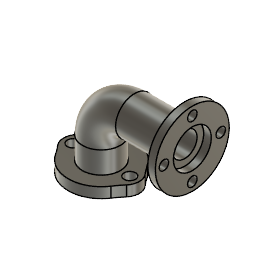
MaRS_Q5_c (Autodesk Fusion 360 design; units mm, degrees)
part number: 2026-05-28-18-50-45-195
Autodesk Fusion 360 part; units mm, degrees
sketch "Sketch1" plane through (0, 0, 0) normal (1, 0, 0) x (0, 1, 0)
sketch "Sketch2" plane through (0, 0, 0) normal (0, 0, 1) x (1, 0, 0)
  circle A0 through (-62, 0, -40) (-81.5, 11.2583, -40) (-81.5, -11.2583, -40)
  arc A1 through (-104.26, -19.2055, -40) (-75, -35, -40) (-45.74, -19.2055, -40)
  arc A2 through (-45.74, 19.2055, -40) (-75, 35, -40) (-104.26, 19.2055, -40)
  arc A3 through (-38.6429, -9.7987, -40) (-35, 0, -40) (-38.6429, 9.7987, -40)
  arc A4 through (-111.0884, 10.1122, -40) (-114.8217, 0, -40) (-111.0884, -10.1122, -40)
  circle A5 through (-55, 0, -40) (-85, 17.3205, -40) (-85, -17.3205, -40)
  arc A6 through (-111.0884, 10.1122, -40) (-107.5304, 14.5508, -40) (-104.26, 19.2055, -40)
  arc A7 through (-104.26, -19.2055, -40) (-107.5304, -14.5508, -40) (-111.0884, -10.1122, -40)
  arc A8 through (-38.6429, -9.7987, -40) (-42.3455, -14.3859, -40) (-45.74, -19.2055, -40)
  arc A9 through (-45.74, 19.2055, -40) (-42.3455, 14.3859, -40) (-38.6429, 9.7987, -40)
  circle A10 through (-39, 0, -40) (-48, 5.1962, -40) (-48, -5.1962, -40)
  circle A11 through (-99, 0, -40) (-108, 5.1962, -40) (-108, -5.1962, -40)
  dimension "d59" = 12
  dimension "d60" = 12
sketch "Sketch3" plane through (0, 0, 0) normal (0, 1, 0) x (1, 0, 0)
sketch "Sketch4" plane through (0, 0, 0) normal (0, 0, 1) x (1, 0, 0)
sketch "Sketch5" plane through (0, 0, 0) normal (0, 1, 0) x (1, 0, 0)
  line L0 (-75, 40) -> (-75, 17)
  line L1 (-40, -18) -> (13, -18)
  arc A0 (-75, 17) -> (-40, -18) centre (-40, 17) ccw
  line L2 (-95, 37.5) -> (-95, 17)
  arc A1 (-95, 17) -> (-40, -38) centre (-40, 17) ccw
  line L3 (-40, -38) -> (10.5, -38)
  line L4 (-75, 40) -> (-75, 17)
  arc A2 (-75, 17) -> (-40, -18) centre (-40, 17) ccw
  line L5 (-40, -18) -> (13, -18)
  line L6 (-55, 37.5) -> (-55, 17)
  arc A3 (-55, 17) -> (-40, 2) centre (-40, 17) ccw
  line L7 (-40, 2) -> (10.5, 2)
  line L8 (-88, 40) -> (-88, 17)
  arc A4 (-88, 17) -> (-40, -31) centre (-40, 17) ccw
  line L9 (-40, -31) -> (13, -31)
  line L10 (-62, 40) -> (-62, 17)
  arc A5 (-62, 17) -> (-40, -5) centre (-40, 17) ccw
  line L11 (-40, -5) -> (13, -5)
  line L12 (13, -40.5) -> (13, -44)
  line L13 (13, 4.5) -> (13, 8)
  arc A6 (10.5, 2) -> (13, 4.5) centre (10.5, 4.5) ccw
  arc A7 (13, -40.5) -> (10.5, -38) centre (10.5, -40.5) ccw
  line L14 (-52.5, 40) -> (-51, 40)
  line L15 (-97.5, 40) -> (-99, 40)
  arc A8 (-95, 37.5) -> (-97.5, 40) centre (-97.5, 37.5) ccw
  arc A9 (-52.5, 40) -> (-55, 37.5) centre (-52.5, 37.5) ccw
  point P0 (-75, -18)
  dimension "d26" = 58
  dimension "d27" = 88
  dimension "d28" = 35
  dimension "d30" = 0
  dimension "d32" = 13
  dimension "d33" = -13
  dimension "d47" = 2.5
  dimension "d48" = 2.5
  dimension "d49" = 2.5
  dimension "d50" = 2.5
  constraint vertical L0
  constraint perpendicular L0 L1
  constraint coincident P0 L0
  constraint coincident P0 L1
  constraint tangent L0 A0
  constraint tangent L1 A0
  constraint perpendicular L3 L12
  constraint perpendicular L7 L13
  constraint concentric A0 A3
  constraint tangent L6 A3
  constraint tangent A3 L7
  constraint tangent L13 A6
  constraint tangent L7 A6
  constraint concentric A0 A1
  constraint tangent L2 A1
  constraint tangent A1 L3
  constraint tangent L3 A7
  constraint tangent L12 A7
  constraint perpendicular L6 L14
  constraint perpendicular L2 L15
  constraint tangent L15 A8
  constraint tangent L2 A8
  constraint tangent L6 A9
  constraint tangent L14 A9
  measures "d26" distance of L0.start P0
  measures "d27" distance of P0 L1.end
  measures "d28" radius of A0
  measures "d47" radius of A6
  measures "d48" radius of A7
  measures "d49" radius of A8
  measures "d50" radius of A9
sketch "Sketch6" plane through (0, 0, 0) normal (1, 0, 0) x (0, 1, 0)
  circle A0 through (39, 18, 13) (-19.5, 51.775, 13) (-19.5, -15.775, 13)
  circle A1 through (20, 18, 13) (-10, 35.3205, 13) (-10, 0.6795, 13)
  circle A2 through (13, 18, 13) (-6.5, 29.2583, 13) (-6.5, 6.7417, 13)
  circle A3 through (5, 48, 13) (-2.5, 52.3301, 13) (-2.5, 43.6699, 13)
  circle A4 through (-25, 18, 13) (-32.5, 22.3301, 13) (-32.5, 13.6699, 13)
  circle A5 through (5, -12, 13) (-2.5, -7.6699, 13) (-2.5, -16.3301, 13)
  circle A6 through (35, 18, 13) (27.5, 22.3301, 13) (27.5, 13.6699, 13)
  dimension "d34" = 78
  dimension "d35" = 40
  dimension "d36" = 26
  dimension "d44" = 10
sketch "Sketch8" plane through (13, 0, 0) normal (1, 0, 0) x (0, 1, 0)
  circle A0 centre (0, 48) radius 5
  dimension "d43" = 10
  measures "d43" diameter of A0
sketch "Sketch9" plane through (0, 0, 0) normal (1, 0, 0) x (0, 1, 0)
sketch "Sketch10" plane through (13, 0, 0) normal (1, 0, 0) x (0, 1, 0)
sweep "Sweep2" add profiles "Sketch6" path "Sketch5" along L0 A0 L1 section 1 contours A1 in plane through (13, 0, 0) normal (1, 0, 0) makes body 1
extrude "Extrude1" add sketch "Sketch6" along normal blind 8 separate body contours A0 in plane through (13, 0, 0) normal (1, 0, 0) makes body 2
extrude "Extrude2" add sketch "Sketch2" against normal blind 11 separate body contours A1 A2 A3 A4 A6 A7 A8 A9 in plane through (0, 0, -40) normal (0, 0, 1) makes body 3
move_body "Move1" bodies 3 1 2 to x (1, 0, 0) y (0, 1, 0) z (0, 0, 1) at (0, 0, 50)
sweep "Sweep1" [rolled back] twist angle 0 taper angle 0
sketch "Sketch7" plane through (0, 0, 0) normal (1, 0, 0) x (0, 1, 0)
